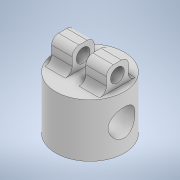
# Autodesk Inventor part: TubeMount
Saved by Autodesk Inventor 2022 (Build 260153000, 153)
## iProperties
Created: 2022-02-12
Part Number: TubeMount
Material: Generic
Document SubType Name: Modeling
Designer: ultra
Density: 1 g/cm^3
Appearance: Default
Author: ultra
Autodesk Inventor part; units mm, degrees
ref_plane "YZ Plane" through (0, 0, 0) normal (1, 0, 0) x (0, 1, 0)
ref_plane "XZ Plane" through (0, 0, 0) normal (0, 1, 0) x (-1, 0, 0)
ref_plane "XY Plane" through (0, 0, 0) normal (0, 0, 1) x (1, 0, 0)
sketch "Sketch1" plane through (0, 0, 0) normal (1, 0, 0) x (0, 1, 0)
  circle A0 centre (0, 0) radius 3.175
  line L0 (-5.08, 5.08) -> (5.08, 5.08)
  line L1 (5.08, 5.08) -> (5.08, -5.08)
  line L2 (5.08, -5.08) -> (-5.08, -5.08)
  line L3 (-5.08, -5.08) -> (-5.08, 5.08)
  line L4 (-5.08, 5.08) -> (5.08, -5.08) construction
  line L5 (5.08, 5.08) -> (-5.08, -5.08) construction
  dimension "d0" = 6.35
  dimension "d1" = 10.16
  dimension "d2" = 10.16
  constraints: 12 end point, 2 midpoint, 2 parallel, 1 centre point, 1 coincident, 1 horizontal, 1 perpendicular
  measures "d0" diameter of A0
  measures "d1" distance of L1.end L2.end
  measures "d2" distance of L0.end L1.end
extrude "Extrusion1" add sketch "Sketch1" along normal blind 12.7
sketch "Sketch2" plane through (0, -5.08, -5.08) normal (0, -1, 0) x (1, 0, 0)
  line L0 (-19.05, 30.48) -> (31.75, 30.48)
  line L1 (31.75, 30.48) -> (31.75, -20.32)
  line L2 (31.75, -20.32) -> (-19.05, -20.32)
  line L3 (-19.05, -20.32) -> (-19.05, 30.48)
  line L4 (-19.05, 30.48) -> (31.75, -20.32) construction
  line L5 (31.75, 30.48) -> (-19.05, -20.32) construction
  circle A0 centre (6.35, 5.08) radius 15.875
  point P0 (0, 5.08)
  dimension "d7" = 50.8
  dimension "d8" = 50.8
  dimension "d9" = 31.75
  constraints: 12 end point, 2 midpoint, 2 parallel, 1 centre point, 1 coincident, 1 horizontal, 1 perpendicular
  measures "d7" distance of L1.end L2.end
  measures "d8" distance of L0.end L1.end
  measures "d9" diameter of A0
extrude "Extrusion2" add sketch "Sketch2" along normal blind 6.35 contours A0
sketch "Sketch3" plane through (0, 5.08, 5.08) normal (0, 1, 0) x (1, 0, 0)
  line L0 (9.525, 17.78) -> (3.175, 17.78)
  line L1 (3.175, 17.78) -> (3.175, -7.62)
  line L2 (3.175, -7.62) -> (9.525, -7.62)
  line L3 (9.525, -7.62) -> (9.525, 17.78)
  line L4 (9.525, 17.78) -> (3.175, -7.62) construction
  line L5 (3.175, 17.78) -> (9.525, -7.62) construction
  point P0 (0, 5.08)
  point P1 (6.35, 5.08)
  dimension "d12" = 6.35
  dimension "d13" = 25.4
  constraints: 12 end point, 2 midpoint, 2 parallel, 1 horizontal, 1 perpendicular
  measures "d12" distance of L2.end L1.end
  measures "d13" distance of L1.end L0.end
extrude "Extrusion3" cut sketch "Sketch3" against normal up to surface (10.16 mm away)
sketch "Sketch5" plane through (12.7, 0, 0) normal (1, 0, 0) x (0, 0, -1)
  line L0 (5.08, -5.08) -> (5.08, 5.08) projected
  line L1 (5.08, 5.08) -> (-5.08, 5.08) projected
  line L2 (-5.08, 5.08) -> (-5.08, -5.08) projected
  line L3 (-5.08, -5.08) -> (5.08, -5.08) projected
  circle A0 centre (0, 0) radius 3.175 projected
extrude "Extrusion4" add sketch "Sketch5" along normal blind 6.35
sketch "Sketch6" plane through (0, 0, 0) normal (-1, 0, 0) x (0, 0, 1)
  line L0 (-5.08, -5.08) -> (-5.08, 5.08) projected
  line L1 (5.08, -5.08) -> (-5.08, -5.08) projected
  line L2 (5.08, 5.08) -> (5.08, -5.08) projected
  line L3 (-5.08, 5.08) -> (5.08, 5.08) projected
  circle A0 centre (0, 0) radius 3.175 projected
extrude "Extrusion5" add sketch "Sketch6" along normal blind 6.35
fillet "Fillet3" radius 3.175 4 edges at (14.2875, 5.08, -5.08) (-1.5875, 5.08, -5.08) (-1.5875, 5.08, 5.08) (14.2875, 5.08, 5.08)
sketch "Sketch10" plane through (6.35, -11.43, 0) normal (0, -1, 0) x (1, 0, 0)
  circle A0 centre (0, 0) radius 15.875 projected
  point P0 (-6.35, 0)
extrude "Extrusion9" add sketch "Sketch10" along normal blind 18.35
sketch "Sketch11" plane through (0, 0, 0) normal (1, 0, 0) x (0, 1, 0)
  line L0 (-29.78, 15.875) -> (-29.78, -15.875) projected
  line L1 (-29.78, 0) -> (-17.4356, 0)
  circle A0 centre (-17.4356, 0) radius 6.2
  point P0 (0, 0)
  dimension "d37" = 12.3444
  dimension "d38" = 12.4
  constraints: 2 end point, 1 centre point, 1 coincident, 1 horizontal, 1 midpoint
  measures "d37" distance of L1.start L1.end
  measures "d38" diameter of A0
extrude "Extrusion10" cut sketch "Sketch11" along normal mid plane 127
fillet "Fillet9" radius 3.175 4 edges at (14.2875, -5.08, -5.08) (-1.5875, -5.08, -5.08) (-1.5875, -5.08, 5.08) (14.2875, -5.08, 5.08)
body "Solid1"
